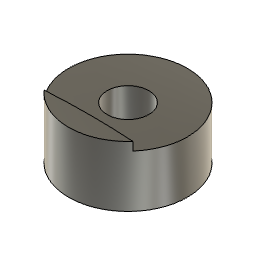
sphere2_dist_back v3 (Autodesk Fusion 360 design; units mm, degrees)
Autodesk Fusion 360 part; units mm, degrees
sketch "Skizze1" plane through (0, 0, 0) normal (0, 0, 1) x (1, 0, 0)
  line L0 (-39.3753, 0) -> (42.4042, 0) construction
  line L1 (0, 170.6208) -> (0, -60) construction
  line L2 (-58.6161, 63) -> (60, 63) construction
  circle A0 centre (0, 63) radius 1.75
  circle A1 centre (0, 63) radius 5
  arc A2 (3.7412, 59.6829) -> (-3.7412, 59.6829) centre (0, 0) ccw
  point P0 (0, 63)
  dimension "d1" = 63
  dimension "d3" = 3.5
  dimension "d4" = 10
  dimension "d5" = 59.8
  constraint horizontal L0
  constraint coincident A2.centre L0
  constraint vertical L1
  constraint coincident A2.centre L1
  constraint horizontal L2
  constraint coincident L1 P0
  constraint coincident L2 P0
  constraint coincident P0 A0.centre
  constraint concentric A0 A1
  constraint coincident A2.centre origin
  constraint coincident A1 A2.end
  constraint coincident A1 A2.start
  measures "d1" distance of A2.centre L2
  measures "d3" diameter of A0
  measures "d4" diameter of A1
  measures "d5" radius of A2
extrude "Extrusion1" add sketch "Skizze1" along normal blind 4.4
extrude "Extrusion2" add sketch "Skizze1" along normal blind 5.1 contours A1 A2 picked at (0, 59.1913)
